Autodesk Fusion 360 part; units mm, degrees
(part 4 of 4)
extrude "Extrude10" cut 1 faces at (-4.0332, 0.2236, 45.5) along direction (0, 0, -1) blind 10 in component "Spur Gear (10 teeth)"
extrude "Extrude11" cut 1 faces at (-4.0332, 0.2236, 35.5) along direction (0, 0, -1) blind 30 in component "Spur Gear (10 teeth)"
extrude "Extrude12" add 1 faces at (-4.0332, 0.2236, 5.5) along direction (0, 0, 1) blind 0.25 in component "Spur Gear (10 teeth)"
component "Spur Gear (10 teeth)" placed x (1, 0, 0) y (0, 1, 0) z (0, 0, 1) at (-0.187, -0.2464, 0.0535)
